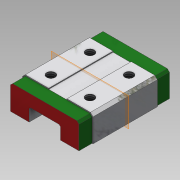
# Autodesk Inventor part: MGN Block
Saved by Autodesk Inventor 2016 (Build 200138000, 138)
## iProperties
Created: 2017-05-18
Part Number: MGN Block
Material: Generic
Document SubType Name: Modeling
Designer: 31745
Density: 1 g/cm^3
Appearance: Aluminum - Dark
Author: 31745
Autodesk Inventor part; units mm, degrees
ref_plane "YZ Plane" through (0, 0, 0) normal (1, 0, 0) x (0, 1, 0)
ref_plane "XZ Plane" through (0, 0, 0) normal (0, 1, 0) x (-1, 0, 0)
ref_plane "XY Plane" through (0, 0, 0) normal (0, 0, 1) x (1, 0, 0)
sketch "Sketch1" plane through (0, 0, 0) normal (0, 0, 1) x (1, 0, 0)
  line L0 (0, 0) -> (27, 0)
  line L1 (27, 0) -> (27, 10)
  line L2 (27, 10) -> (0, 10)
  line L3 (0, 10) -> (0, 0)
  line L4 (7.5, 0) -> (19.5, 0)
  line L5 (19.5, 0) -> (19.5, 5)
  line L6 (19.5, 5) -> (7.5, 5)
  line L7 (7.5, 5) -> (7.5, 0)
  point P0 (13.5, 5)
  point P1 (13.5, 10)
  dimension "d0" = 27
  dimension "d1" = 10
  dimension "d2" = 5
  dimension "d3" = 12
  constraints: 16 end point, 4 parallel, 2 horizontal, 2 midpoint, 2 perpendicular, 1 point on line, 1 vertical alignment
  measures "d0" distance of L2.end L1.end
  measures "d1" distance of L1.end L0.end
  measures "d2" distance of L4.end L5.end
  measures "d3" distance of L5.end L6.end
extrude "Extrusion1" add sketch "Sketch1" along normal blind 34.7 contours L3 L2 L1 L0 L5 L6 L7
chamfer "Chamfer1" distance 1 angle 45 2 edges at (27, 10, 17.35) (0, 10, 17.35)
chamfer "Chamfer2" distance 0.5 angle 45 2 edges at (7.5, 5, 17.35) (19.5, 5, 17.35)
sketch "Sketch2" plane through (1, 10, 0) normal (0, 1, 0) x (1, 0, 0)
  line L0 (18, -34.7) -> (18, 0) projected
  line L1 (-1, 0) -> (-1, -34.7) projected
  line L2 (25, 0) -> (0, 0) projected
  line L3 (5, -9.85) -> (20, -9.85)
  line L4 (20, -9.85) -> (20, -24.85)
  line L5 (20, -24.85) -> (5, -24.85)
  line L6 (5, -24.85) -> (5, -9.85)
  line L7 (25, 0) -> (25, -34.7) projected
  point P0 (-1, -17.35)
  point P1 (12.5, 0)
  point P2 (12.5, -9.85)
  point P3 (12.5, 0)
  point P4 (20, -17.35)
  point P5 (25, -17.35)
  dimension "d12" = 15
  dimension "d13" = 15
  constraints: 8 end point, 6 midpoint, 4 coincident, 2 parallel, 1 horizontal, 1 horizontal alignment, 1 perpendicular, 1 vertical alignment
  measures "d12" distance of L3.end L4.end
  measures "d13" distance of L3.start L3.end
hole "Hole1" at (21, 10, 9.85) at (21, 10, 24.85) at (6, 10, 24.85) at (6, 10, 9.85) direction (0, -1, 0) diameter 3.242 depth 5 tip angle 118 thread size "M4x0.7" class "6H" standard "ISO Metric profile"
sketch "Sketch3" plane through (0, 0, 34.7) normal (0, 0, 1) x (1, 0, 0)
  line L0 (0, 9) -> (0, 0) projected
  line L1 (0, 9) -> (1, 10) projected
  line L2 (26, 10) -> (1, 10) projected
  line L3 (26, 10) -> (27, 9) projected
  line L4 (27, 0) -> (27, 9) projected
  line L5 (0.375, 0) -> (0.375, 8.8447)
  line L6 (0.375, 8.8447) -> (1.1553, 9.625)
  line L7 (1.1553, 9.625) -> (25.8447, 9.625)
  line L8 (25.8447, 9.625) -> (26.625, 8.8447)
  line L9 (26.625, 8.8447) -> (26.625, 0)
  line L10 (19.5, 0) -> (27, 0) projected
  line L11 (26.625, 0) -> (27, 0)
  line L12 (27, 0) -> (0.375, 0)
  line L13 (0, 0) -> (7.5, 0) projected
  line L14 (0.375, 0) -> (0, 0)
  dimension "d21" = 0.375
  constraints: 16 end point, 2 collinear, 1 horizontal, 4 other
  measures "d21" distance between parallel lines of L2 L7
extrude "Extrusion2" cut sketch "Sketch3" against normal blind 5 contours L1 L2 L3 L4 L10 L9 L8 L7 L6 L5 L13 L0
ref_plane "Work Plane1" through (0, 0, 17.35) normal (0, 0, 1) x (1, 0, 0)
mirror "Mirror1" about plane through (0, 0, 17.35) normal (0, 0, 1) of "Extrusion2"
sketch "Sketch4" plane through (1, 10, 29.7) normal (0, 1, 0) x (1, 0, 0)
  circle A0 centre (5, 19.85) radius 1.621 projected
  circle A1 centre (20, 4.85) radius 1.621 projected
  circle A2 centre (20, 19.85) radius 1.621 projected
  circle A3 centre (5, 4.85) radius 1.621 projected
  line L0 (25, 24.7) -> (0, 24.7) projected
  line L1 (0, 0) -> (0, 24.7) projected
  line L2 (0, 0) -> (25, 0) projected
  line L3 (25, 24.7) -> (25, 0) projected
  line L4 (25, 24.7) -> (0, 24.7) projected
  line L5 (0, 0) -> (25, 0) projected
  line L6 (9, 24.7) -> (16, 24.7)
  line L7 (16, 24.7) -> (16, 0)
  line L8 (16, 0) -> (9, 0)
  line L9 (9, 0) -> (9, 24.7)
  point P0 (-1, 29.7)
  point P1 (12.5, 24.7)
  point P2 (12.5, 24.7)
  dimension "d24" = 7
  constraints: 8 end point, 2 midpoint, 2 parallel, 2 point on line, 1 coincident, 1 horizontal, 1 perpendicular
  measures "d24" distance between parallel lines of L7 L9
extrude "Extrusion3" cut sketch "Sketch4" against normal blind 0.35 contours L7 L2 L9 L0
body "Solid1"
